Crank Disk OLD (Autodesk Fusion 360 design; units mm, degrees)
Autodesk Fusion 360 part; units mm, degrees
sketch "Sketch1" plane through (0, 0, 0) normal (1, 0, 0) x (0, 1, 0)
  circle A0 centre (0, 0) radius 3.2
  circle A1 centre (0, 0) radius 35
  circle A2 centre (0, 0) radius 25 construction
  circle A3 centre (23.0759, 9.6178) radius 3.2
  dimension "d1" = 6.4
  dimension "d2" = 70
  dimension "d3" = 50
  dimension "d4" = 6.4
  constraint coincident A0.centre A1.centre
  constraint concentric A1 A2
  constraint coincident A2 A3.centre
  measures "d1" diameter of A0
  measures "d2" diameter of A1
  measures "d3" diameter of A2
  measures "d4" diameter of A3
extrude "Extrude1" add sketch "Sketch1" along normal blind 15
